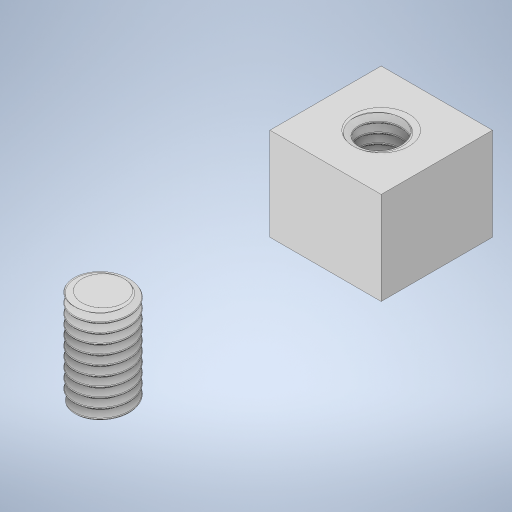
# Autodesk Inventor part: Sample
Saved by Autodesk Inventor 2024 (Build 280153000, 153)
## iProperties
Created: 2024-01-02
Part Number: Sample
Material: Generic
Document SubType Name: Modeling
Designer: Admin
Density: 1 g/cm^3
Appearance: Default
VLDS_Profile: Default Part
VLDS_TimeStamp: 2024-01-02
VLDS_FailCnt: 0
VLDS_AcceptCnt: 0
Author: Admin
Autodesk Inventor part; units mm, degrees
ref_plane "YZ Plane" through (0, 0, 0) normal (1, 0, 0) x (0, 1, 0)
ref_plane "XZ Plane" through (0, 0, 0) normal (0, 1, 0) x (-1, 0, 0)
ref_plane "XY Plane" through (0, 0, 0) normal (0, 0, 1) x (1, 0, 0)
sketch "Sketch1" plane through (0, 0, 0) normal (0, 0, 1) x (1, 0, 0)
  circle A0 centre (0, 0) radius 3
  line L0 (0, 0) -> (0, 30)
  circle A1 centre (0, 30) radius 3
  line L1 (0, 30) -> (0, 24)
  line L2 (0, 24) -> (-6, 24)
  line L3 (0, 24) -> (6, 24)
  line L4 (6, 24) -> (6, 36)
  line L5 (6, 36) -> (-6, 36)
  line L6 (-6, 36) -> (-6, 24)
  dimension "d0" = 6
  dimension "d9" = 30
  dimension "d10" = 6
  dimension "d11" = 6
  dimension "d12" = 6
  dimension "d13" = 6
  dimension "d14" = 12
  constraints: 14 end point, 4 perpendicular, 2 centre point, 2 coincident, 1 horizontal, 1 point on line, 1 vertical
  measures "d0" diameter of A0
  measures "d9" distance of L0.start L0.end
  measures "d10" diameter of A1
  measures "d11" distance of L1.start L1.end
  measures "d12" distance of L1.end L2.end
  measures "d13" distance of L1.end L3.end
  measures "d14" distance of L3.end L4.end
extrude "Extrusion1" add sketch "Sketch1" along normal blind 10
thread "Thread1" size "M6x1" class "6g" standard "ANSI Metric M Profile" length 38.1
thread "Thread2" size "M6x1" class "6H" standard "ANSI Metric M Profile" length 38.1
sketch "Sketch3" plane through (0, 0, 10) normal (-1, 0, 0) x (0, 1, 0)
  line L0 (3, 0) -> (3, 38.1)
  line L1 (3, 38.1) -> (2.2585, 38.1)
  line L2 (2.2585, 38.1) -> (2.2585, 0)
  line L3 (2.2585, 0) -> (3, 0)
  line L4 (0, -8.9286) -> (0, 45.9381) projected
  constraints: 8 end point
revolve "Revolution1" cut sketch "Sketch3" angle 360 about axis through (0, 0, 10) along (0, 0, -1)
sketch "Sketch4" plane through (0, 0, 10) normal (-1, 0, 0) x (0, 1, 0)
  line L0 (3, 38.1) -> (2.2585, 38.1)
  line L1 (2.2585, 0) -> (3, 0)
  line L2 (0, -8.9286) -> (0, 45.9381) projected
  line L3 (2.2585, 10) -> (-2.2585, 10) projected
  line L4 (3, 10) -> (2.2585, 10)
  line L5 (2.2585, 10) -> (2.2585, 0)
  line L6 (2.2585, 0) -> (3, 0)
  line L7 (3, 0) -> (3, 10)
  line L8 (2.2585, 10) -> (2.2585, 23.9286)
  line L9 (2.2585, 23.9286) -> (3, 23.9286)
  line L10 (3, 23.9286) -> (3, 10)
  constraints: 18 end point, 3 perpendicular, 2 parallel, 1 horizontal, 1 vertical
revolve "Revolution2" add sketch "Sketch4" angle 360 about axis through (0, 0, 10) along (0, 0, -1) separate body contours L5 L4 L7 L1
sketch "Sketch2" plane through (0, 0, 10) normal (1, 0, 0) x (0, 0, -1)
  line L0 (-0.5834, -2.3093) -> (-0.5001, -2.3093) construction
  line L1 (0.0832, -2.9496) -> (-0.0001, -3.1097) construction
  line L2 (-1.0001, -3.1097) -> (-1.0834, -2.9496) construction
  line L3 (-0.4168, -2.3093) -> (-0.5001, -2.1492) construction
  line L4 (-0.5001, -2.1492) -> (-0.5834, -2.3093) construction
  line L5 (-1.0001, -3.1097) -> (-0.9168, -2.9496) construction
  line L6 (-0.4168, -2.3093) -> (-0.0834, -2.9496)
  line L7 (-1.0834, -2.9496) -> (-0.9168, -2.9496) construction
  arc A0 (-1.0834, -2.9496) -> (-1.0001, -3.0002) centre (-1.0001, -2.9062) ccw construction
  line L8 (0.0832, -2.9496) -> (-0.0834, -2.9496) construction
  line L9 (-1.0001, -3.1097) -> (-1.0001, -2.9496) construction
  line L10 (-0.0001, -3.1097) -> (-0.0001, -2.9496) construction
  line L11 (-0.5001, -2.1492) -> (-0.5001, -2.2587) construction
  line L12 (-1.0001, -3.0002) -> (-0.0001, -3.0002)
  arc A1 (-1.0001, -3.0002) -> (-0.9168, -2.9496) centre (-1.0001, -2.9062) ccw
  line L13 (-0.0834, -2.9496) -> (-0.0001, -3.1097) construction
  line L14 (-0.9168, -2.9496) -> (-0.5834, -2.3093)
  line L15 (-0.0001, -0.0002) -> (-0.0001, 0.0177)
  line L16 (-0.0001, 0.0177) -> (-0.0001, -0.0002)
  line L17 (-0.0001, -0.0002) -> (0.0334, -0.0002)
  arc A2 (-0.0834, -2.9496) -> (-0.0001, -3.0002) centre (-0.0001, -2.9062) ccw
  arc A3 (-0.0001, -3.0002) -> (0.0832, -2.9496) centre (-0.0001, -2.9062) ccw construction
  arc A4 (-0.5001, -2.2587) -> (-0.5834, -2.3093) centre (-0.5001, -2.3527) ccw
  arc A5 (-0.4168, -2.3093) -> (-0.5001, -2.2587) centre (-0.5001, -2.3527) ccw
  line L18 (-0.5001, -2.2587) -> (-0.5001, -2.3093) construction
  line L19 (-0.5001, -2.3093) -> (-0.4168, -2.3093) construction
  dimension "d19" = 55
  dimension "d20" = 0.1601
  dimension "d21" = 0.1601
  dimension "Sketch2_ThreadOffset" = 0
  dimension "Sketch2_MajorRadius" = 3
  dimension "d24" = 1
  dimension "Sketch2_MinorRadius" = 2.2585
  constraints: 40 end point, 12 point on circle, 10 parallel, 8 tangent, 6 centre point, 6 collinear, 2 midpoint, 2 point on line, 1 horizontal, 1 perpendicular, 3 other
  measures "d19" angle of L6 L14
  measures "d20" distance of L3.end L0.end
  measures "d21" distance of L1.end L10.end
  measures "Sketch2_ThreadOffset" distance between parallel lines of L15 L10
  measures "Sketch2_MajorRadius" distance from line of L12 L15.start
  measures "d24" distance from line of L1.end L9
  measures "Sketch2_MinorRadius" distance edge to line of A5 L17
coil "Coil1" sketch "Sketch2" operation cut axis through (0, 0, 10) along (0, 0, -1) pitch 1.001 turns 40.05994 hand right bodies 2
sketch "Sketch6" plane through (0, 30, 10) normal (-1, 0, 0) x (0, 1, 0)
  line L0 (3, 38.1) -> (2.2585, 38.1)
  line L1 (2.2585, 0) -> (3, 0)
  line L2 (0, -8.9953) -> (0, 46.3381) projected
  line L3 (6, 10) -> (-6, 10) projected
  line L4 (0, 10) -> (3, 10)
  line L5 (0, 0) -> (3, 0)
  line L6 (3, 10) -> (2.2585, 10)
  line L7 (2.2585, 10) -> (2.2585, 0)
  line L8 (2.2585, 0) -> (3, 0)
  line L9 (3, 0) -> (3, 10)
  constraints: 16 end point, 3 parallel, 2 point on line, 1 horizontal, 1 midpoint, 1 perpendicular
revolve "Revolution3" add sketch "Sketch6" angle 360 about axis through (0, 30, 10) along (0, 0, -1) separate body contours L7 L3 L9 L1
sketch "Sketch5" plane through (0, 33, 10) normal (1, 0, 0) x (0, 0, -1)
  line L0 (-0.5834, -0.0507) -> (-0.5001, -0.0507) construction
  line L1 (0.0832, -0.6911) -> (-0.0001, -0.8511) construction
  line L2 (-1.0001, -0.8511) -> (-1.0834, -0.6911) construction
  line L3 (-0.4168, -0.0507) -> (-0.5001, 0.1093) construction
  line L4 (-0.5001, 0.1093) -> (-0.5834, -0.0507) construction
  line L5 (-1.0001, -0.8511) -> (-0.9168, -0.6911) construction
  line L6 (-0.4168, -0.0507) -> (-0.0834, -0.6911)
  line L7 (-1.0834, -0.6911) -> (-0.9168, -0.6911) construction
  arc A0 (-1.0834, -0.6911) -> (-1.0001, -0.7416) centre (-1.0001, -0.6477) ccw construction
  line L8 (0.0832, -0.6911) -> (-0.0834, -0.6911) construction
  line L9 (-1.0001, -0.8511) -> (-1.0001, -0.6911) construction
  line L10 (-0.0001, -0.8511) -> (-0.0001, -0.6911) construction
  line L11 (-0.5001, 0.1093) -> (-0.5001, -0.0002) construction
  line L12 (-1.0001, -0.7416) -> (-0.0001, -0.7416)
  arc A1 (-1.0001, -0.7416) -> (-0.9168, -0.6911) centre (-1.0001, -0.6477) ccw
  line L13 (-0.0834, -0.6911) -> (-0.0001, -0.8511) construction
  line L14 (-0.9168, -0.6911) -> (-0.5834, -0.0507)
  line L15 (-0.0001, -0.0002) -> (-0.0001, 0.0177)
  line L16 (-0.0001, 0.0177) -> (-0.0001, -0.0002)
  line L17 (-0.0001, -0.0002) -> (0.0334, -0.0002)
  arc A2 (-0.0834, -0.6911) -> (-0.0001, -0.7416) centre (-0.0001, -0.6477) ccw
  arc A3 (-0.0001, -0.7416) -> (0.0832, -0.6911) centre (-0.0001, -0.6477) ccw construction
  arc A4 (-0.5001, -0.0002) -> (-0.5834, -0.0507) centre (-0.5001, -0.0941) ccw
  arc A5 (-0.4168, -0.0507) -> (-0.5001, -0.0002) centre (-0.5001, -0.0941) ccw
  line L18 (-0.5001, -0.0002) -> (-0.5001, -0.0507) construction
  line L19 (-0.5001, -0.0507) -> (-0.4168, -0.0507) construction
  dimension "d38" = 55
  dimension "d39" = 0.1601
  dimension "d40" = 0.1601
  dimension "Sketch5_ThreadOffset" = 0
  dimension "Sketch5_MajorRadius" = 0.7415
  dimension "d43" = 1
  dimension "Sketch5_MinorRadius" = 0
  constraints: 40 end point, 12 point on circle, 10 parallel, 8 tangent, 6 centre point, 6 collinear, 2 midpoint, 2 point on line, 1 horizontal, 1 perpendicular, 3 other
  measures "d38" angle of L6 L14
  measures "d39" distance of L3.end L0.end
  measures "d40" distance of L1.end L10.end
  measures "Sketch5_ThreadOffset" distance between parallel lines of L15 L10
  measures "Sketch5_MajorRadius" distance from line of L12 L15.start
  measures "d43" distance from line of L1.end L9
  measures "Sketch5_MinorRadius" distance edge to line of A5 L17
coil "Coil2" sketch "Sketch5" operation cut axis through (0, 30, 10) along (0, 0, -1) pitch 1.001 turns 40.05994 hand right bodies 3
equation "\"d19\" = d26"
equation "\"d20\" = 0.160083 * Sketch2_Pitch"
equation "\"d21\" = 0.160083 * Sketch2_Pitch"
equation "\"d24\" = Sketch2_Pitch"
equation "\"d38\" = d45"
equation "\"d39\" = 0.160083 * Sketch5_Pitch"
equation "\"d40\" = 0.160083 * Sketch5_Pitch"
equation "\"d43\" = Sketch5_Pitch"
equation "\"d26\" = 55deg"
equation "\"Sketch2_Pitch\" = 1"
equation "\"d45\" = 55deg"
equation "\"Sketch5_Pitch\" = 1"
body "Solid1"
body "Solid2"
body "Solid3"
